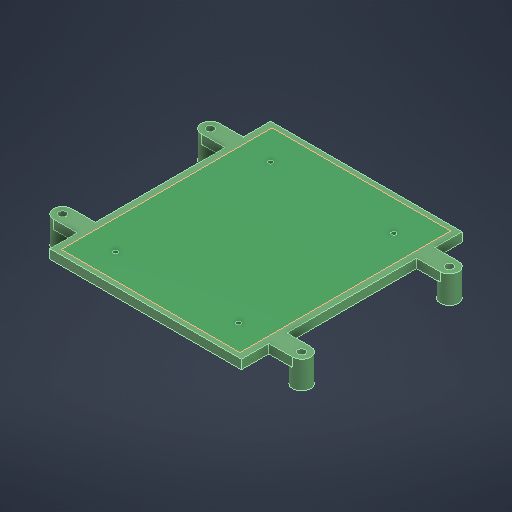
# Autodesk Inventor part: PCB_Gehaeuse_o
Saved by Autodesk Inventor 2026.2 (Build 302298000, 298)
## iProperties
Created: 2026-01-10
Part Number: PCB_Gehaeuse_o
Material: Generisch
Document SubType Name: Modeling
Designer: Alex
Density: 1 g/cm^3
Appearance: Vorgabe
Author: Alex
Autodesk Inventor part; units mm, degrees
ref_plane "YZ Plane" through (0, 0, 0) normal (1, 0, 0) x (0, 1, 0)
ref_plane "XZ Plane" through (0, 0, 0) normal (0, 1, 0) x (-1, 0, 0)
ref_plane "XY Plane" through (0, 0, 0) normal (0, 0, 1) x (1, 0, 0)
ref_plane "Arbeitsebene1" through (145, 129, -5.4115) normal (0, 0, -1) x (-1, 0, 0)
sketch "Skizze1" plane through (145, 129, -5.4115) normal (0, 0, -1) x (-1, 0, 0)
  line L0 (0, -105) -> (89, -105) projected
  line L1 (89, -105) -> (89, 0) projected
  line L2 (0, 0) -> (0, -105) projected
  line L3 (89, 0) -> (0, 0) projected
  line L4 (89, -105) -> (0, 0)
  line L5 (0, -105) -> (89, 0)
  line L6 (97, 8) -> (-8, 8)
  line L7 (-8, 8) -> (-8, -113)
  line L8 (-8, -113) -> (97, -113)
  line L9 (97, -113) -> (97, 8)
  line L10 (97, 8) -> (-8, -113) construction
  line L11 (-8, 8) -> (97, -113) construction
  point P0 (145, -129)
  point P1 (44.5, -52.5)
  dimension "d1" = 105
  dimension "d2" = 121
  constraints: 16 end point, 3 midpoint, 2 parallel, 1 horizontal, 1 perpendicular
  measures "d1" distance of L8.end L7.end
  measures "d2" distance of L7.end L6.end
extrude "Extrusion1" add sketch "Skizze1" along normal blind 5 contours L5 L4 L0 | L2 L4 L5 | L4 L5 L1 | L3 L5 L4 | L9 L8 L7 L6
sketch "Skizze3" plane through (145, 129, -10.4115) normal (0, 0, -1) x (-1, 0, 0)
  circle A0 centre (10, -96.5) radius 1 projected
  circle A1 centre (10, -11.5) radius 1 projected
  circle A2 centre (77.5, -96.5) radius 1 projected
  circle A3 centre (77.5, -11.5) radius 1 projected
  circle A4 centre (77.5, -11.5) radius 4 projected
  circle A5 centre (77.5, -11.5) radius 1.25
  circle A6 centre (77.5, -96.5) radius 4 projected
  circle A7 centre (77.5, -96.5) radius 1.25
  circle A8 centre (10, -96.5) radius 1.25
  circle A9 centre (10, -11.5) radius 1.25
  point P0 (145, -129)
  dimension "d12" = 2.5
  dimension "d13" = 2.5
  dimension "d14" = 2.5
  dimension "d15" = 2.5
  constraints: 4 centre point, 4 coincident
  measures "d12" diameter of A5
  measures "d13" diameter of A7
  measures "d14" diameter of A8
  measures "d15" diameter of A9
extrude "Extrusion3" cut sketch "Skizze3" against normal blind 25.25 contours A0 | A1 | A2 | A3 | A5 | A7 | A8 | A9
sketch "Skizze5" plane through (48, 16, -5.4115) normal (-1, 0, 0) x (0, 0, 1)
  line L0 (0, 0) -> (0, 121) projected
  line L1 (0, 121) -> (-5, 121) projected
  line L2 (-5, 0) -> (-5, 121) projected
  line L3 (0, 0) -> (-5, 0) projected
  line L4 (0, 121) -> (0, 106)
  line L5 (0, 0) -> (0, 15)
  line L6 (0, 106) -> (-5, 106)
  line L7 (-5, 106) -> (-5, 96)
  line L8 (-5, 96) -> (0, 96)
  line L9 (0, 96) -> (0, 106)
  line L10 (0, 15) -> (-5, 15)
  line L11 (-5, 15) -> (-5, 25)
  line L12 (-5, 25) -> (0, 25)
  line L13 (0, 25) -> (0, 15)
  point P0 (5.4115, -16)
  dimension "d24" = 15
  dimension "d25" = 15
  dimension "d26" = 10
  dimension "d27" = 10
  constraints: 20 end point, 4 parallel, 4 point on line, 2 horizontal, 2 perpendicular
  measures "d24" distance of L0.end L4.end
  measures "d25" distance of L0.start L5.end
  measures "d26" distance of L7.end L6.end
  measures "d27" distance of L10.end L11.end
extrude "Extrusion5" add sketch "Skizze5" along normal blind 18 contours L10 L2 L12 L0 | L8 L2 L6 L0
fillet "Rundung1" radius 5 4 edges at (30, 122, -7.9115) (30, 112, -7.9115) (30, 41, -7.9115) (30, 31, -7.9115)
sketch "Skizze6" plane through (153, 16, -5.4115) normal (1, 0, 0) x (0, 0, -1)
  line L0 (0, 121) -> (0, 0) projected
  line L1 (0, 0) -> (5, 0) projected
  line L2 (5, 121) -> (5, 0) projected
  line L3 (0, 121) -> (5, 121) projected
  line L4 (0, 0) -> (0, 15) projected
  line L5 (0, 0) -> (0, 15)
  line L6 (0, 121) -> (0, 106)
  line L7 (0, 15) -> (5, 15)
  line L8 (5, 15) -> (5, 25)
  line L9 (5, 25) -> (0, 25)
  line L10 (0, 25) -> (0, 15)
  line L11 (0, 96) -> (5, 96) projected
  line L12 (0, 106) -> (5, 106)
  line L13 (5, 106) -> (5, 96)
  line L14 (5, 96) -> (0, 96)
  line L15 (0, 96) -> (0, 106)
  point P0 (-5.4115, -16)
  dimension "d31" = 15
  dimension "d32" = 15
  dimension "d33" = 10
  dimension "d34" = 10
  constraints: 20 end point, 4 parallel, 2 horizontal, 2 perpendicular, 2 point on line, 1 collinear
  measures "d31" distance of L0.end L4.end
  measures "d32" distance of L0.start L6.end
  measures "d33" distance of L8.end L7.end
  measures "d34" distance of L12.end L11.end
extrude "Extrusion6" add sketch "Skizze6" along normal blind 18 contours L12 L2 L11 L0 | L9 L2 L7 L0
fillet "Rundung2" radius 5 4 edges at (171, 112, -7.9115) (171, 122, -7.9115) (171, 31, -7.9115) (171, 41, -7.9115)
sketch "Skizze7" plane through (145, 129, -5.4115) normal (0, 0, 1) x (1, 0, 0)
  arc A0 (21, -98) -> (21, -88) centre (21, -93) ccw projected
  line L0 (8, -88) -> (21, -88) projected
  line L1 (8, -17) -> (8, -88) projected
  line L2 (8, -17) -> (21, -17) projected
  arc A1 (21, -17) -> (21, -7) centre (21, -12) ccw projected
  line L3 (8, -7) -> (21, -7) projected
  line L4 (8, 8) -> (8, -7) projected
  line L5 (-97, 8) -> (8, 8) projected
  line L6 (-97, -7) -> (-97, 8) projected
  line L7 (-97, -7) -> (-110, -7) projected
  arc A2 (-110, -7) -> (-110, -17) centre (-110, -12) ccw projected
  line L8 (-97, -17) -> (-110, -17) projected
  line L9 (-97, -88) -> (-97, -17) projected
  line L10 (-97, -88) -> (-110, -88) projected
  arc A3 (-110, -88) -> (-110, -98) centre (-110, -93) ccw projected
  line L11 (-97, -98) -> (-110, -98) projected
  line L12 (-97, -113) -> (-97, -98) projected
  line L13 (8, -113) -> (-97, -113) projected
  line L14 (8, -98) -> (8, -113) projected
  line L15 (8, -98) -> (21, -98) projected
  circle A4 centre (-110, -12) radius 2.1
  circle A5 centre (21, -12) radius 2.1
  circle A6 centre (21, -93) radius 2.1
  arc A7 (-110, -88) -> (-110, -98) centre (-110, -93) ccw projected
  circle A8 centre (-110, -93) radius 2.1
  point P0 (-145, -129)
  dimension "d38" = 4.2
  dimension "d39" = 4.2
  dimension "d40" = 4.2
  dimension "d41" = 4.2
  constraints: 4 centre point, 4 coincident
  measures "d38" diameter of A4
  measures "d39" diameter of A5
  measures "d40" diameter of A6
  measures "d41" diameter of A8
extrude "Extrusion7" cut sketch "Skizze7" against normal blind 18 contours A4 | A5 | A6 | A8
sketch "Skizze8" plane through (145, 129, -10.4115) normal (0, 0, -1) x (-1, 0, 0)
  circle A0 centre (-21, -93) radius 2.1 projected
  circle A1 centre (-21, -12) radius 2.1 projected
  circle A2 centre (110, -93) radius 2.1 projected
  circle A3 centre (110, -12) radius 2.1 projected
  arc A4 (-21, -88) -> (-21, -98) centre (-21, -93) ccw projected
  line L0 (-8, -98) -> (-21, -98) projected
  line L1 (-8, -98) -> (-8, -113) projected
  line L2 (-8, -113) -> (97, -113) projected
  line L3 (97, -113) -> (97, -98) projected
  line L4 (97, -98) -> (110, -98) projected
  arc A5 (110, -98) -> (110, -88) centre (110, -93) ccw projected
  line L5 (97, -88) -> (110, -88) projected
  line L6 (97, -88) -> (97, -17) projected
  line L7 (97, -17) -> (110, -17) projected
  arc A6 (110, -17) -> (110, -7) centre (110, -12) ccw projected
  line L8 (97, -7) -> (110, -7) projected
  line L9 (97, -7) -> (97, 8) projected
  line L10 (97, 8) -> (-8, 8) projected
  line L11 (-8, 8) -> (-8, -7) projected
  line L12 (-8, -7) -> (-21, -7) projected
  arc A7 (-21, -7) -> (-21, -17) centre (-21, -12) ccw projected
  line L13 (-8, -17) -> (-21, -17) projected
  line L14 (-8, -17) -> (-8, -88) projected
  line L15 (-8, -88) -> (-21, -88) projected
  circle A8 centre (-21, -93) radius 5
  circle A9 centre (-21, -12) radius 5
  circle A10 centre (110, -12) radius 5
  circle A11 centre (110, -93) radius 5
  line L16 (97, -113) -> (-8, 8)
  circle A12 centre (44.5, -52.5) radius 10
  point P0 (145, -129)
  dimension "d44" = 20
  constraints: 5 centre point, 4 coincident, 2 end point, 1 concentric, 1 midpoint
  measures "d44" diameter of A12
extrude "Extrusion8" add sketch "Skizze8" along normal blind 10 contours A8 A4 | A7 A9 | A12 L16 | L16 A12 | A11 A5 | A6 A10
